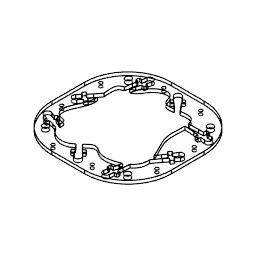
MidPlateShellBearing_v33 (Autodesk Fusion 360 design; units mm, degrees)
Autodesk Fusion 360 part; units mm, degrees
(part 1 of 2)
sketch "Sketch1" plane through (0, 0, 0) normal (0, 0, 1) x (1, 0, 0)
  line L0 (-33.4, -17.4) -> (-33.4, 33.4) construction
  line L1 (-33.4, 33.4) -> (-27.4, 33.4) construction
  line L2 (-33.4, -17.4) -> (-36.4, -17.4)
  line L3 (-36.4, -17.4) -> (-36.4, -27.4)
  line L4 (-36.4, -27.4) -> (-33.4, -27.4)
  line L5 (-33.4, -27.4) -> (-33.4, -17.4)
  line L6 (-27.4, 33.4) -> (-17.4, 33.4)
  line L7 (-17.4, 33.4) -> (-17.4, 36.4)
  line L8 (-17.4, 36.4) -> (-27.4, 36.4)
  line L9 (-27.4, 36.4) -> (-27.4, 33.4)
  line L10 (-17.4, 33.4) -> (33.4, 33.4) construction
  line L11 (33.4, 33.4) -> (33.4, 27.4) construction
  line L12 (33.4, 27.4) -> (36.4, 27.4)
  line L13 (36.4, 27.4) -> (36.4, 17.4)
  line L14 (36.4, 17.4) -> (33.4, 17.4)
  line L15 (33.4, 17.4) -> (33.4, 27.4)
  line L16 (33.4, 17.4) -> (33.4, -33.4) construction
  line L17 (33.4, -33.4) -> (27.4, -33.4) construction
  line L18 (27.4, -33.4) -> (17.4, -33.4)
  line L19 (17.4, -33.4) -> (17.4, -36.4)
  line L20 (17.4, -36.4) -> (27.4, -36.4)
  line L21 (27.4, -36.4) -> (27.4, -33.4)
  line L22 (17.4, -33.4) -> (-33.4, -33.4) construction
  line L23 (-33.4, -33.4) -> (-33.4, -27.4) construction
  line L24 (33.4, 33.4) -> (-33.4, -33.4) construction
  line L25 (33.4, -33.4) -> (-33.4, 33.4) construction
  line L26 (55, -55) -> (-55, -55)
  line L27 (-55, -55) -> (-55, 55)
  line L28 (-55, 55) -> (55, 55)
  line L29 (55, 55) -> (55, -55)
  line L30 (55, -55) -> (-55, 55) construction
  line L31 (-55, -55) -> (55, 55) construction
  line L32 (-34.9, -17.4) -> (-34.9, -7.75) construction
  line L33 (-34.9, -7.75) -> (-38.15, -7.75) construction
  circle A0 centre (-38.15, -7.75) radius 1.25
  line L34 (-34.9, -27.4) -> (-34.9, -38.15) construction
  line L35 (-34.9, -38.15) -> (-37.75, -38.15) construction
  circle A1 centre (-37.75, -38.15) radius 1.25
  circle A2 centre (38.15, -37.75) radius 1.25
  circle A3 centre (7.75, -38.15) radius 1.25
  circle A4 centre (37.75, 38.15) radius 1.25
  circle A5 centre (38.15, 7.75) radius 1.25
  circle A6 centre (-38.15, 37.75) radius 1.25
  circle A7 centre (-7.75, 38.15) radius 1.25
  constraint vertical L0
  constraint perpendicular L0 L1
  constraint horizontal L2
  constraint vertical L3
  constraint horizontal L4
  constraint vertical L5
  constraint horizontal L6
  constraint vertical L7
  constraint horizontal L8
  constraint vertical L9
  constraint perpendicular L7 L10
  constraint perpendicular L10 L11
  constraint horizontal L12
  constraint vertical L13
  constraint horizontal L14
  constraint vertical L15
  constraint perpendicular L14 L16
  constraint perpendicular L16 L17
  constraint horizontal L18
  constraint vertical L19
  constraint horizontal L20
  constraint vertical L21
  constraint perpendicular L19 L22
  constraint coincident origin L24
  constraint coincident origin L25
  constraint horizontal L26
  constraint perpendicular L26 L27
  constraint parallel L26 L28
  constraint parallel L27 L29
  constraint coincident L30 origin
  constraint coincident L31 origin
  constraint midpoint L2 L32.start
  constraint perpendicular L2 L32
  constraint perpendicular L32 L33
  constraint coincident L33.end A0.centre
  constraint midpoint L4 L34.start
  constraint perpendicular L4 L34
  constraint perpendicular L34 L35
  constraint coincident L35.end A1.centre
  measures "d1" distance of L0.start L0.end
  measures "d2" distance of L0.end L1.end
  measures "d3" distance of L0.start L2.end
  measures "d4" distance of L0.start L4.end
  measures "d5" distance of L1.end L6.end
  measures "d6" distance of L1.end L8.end
  measures "d7" distance of L6.end L10.end
  measures "d8" distance of L10.end L11.end
  measures "d9" distance of L11.end L12.end
  measures "d10" distance of L11.end L14.end
  measures "d11" distance of L14.end L16.end
  measures "d12" distance of L16.end L17.end
  measures "d13" distance of L17.end L18.end
  measures "d14" distance of L17.end L20.end
  measures "d15" distance of L18.end L22.end
  measures "d16" distance of L27.end L28.end
  measures "d17" distance of L26.end L27.end
  measures "d22" distance of L32.start L32.end
  measures "d23" distance of L32.end L33.end
  measures "d24" diameter of A0
  measures "d25" distance of L34.start L34.end
  measures "d26" distance of L34.end L35.end
  measures "d27" diameter of A1
extrude "Extrude1" add sketch "Sketch1" along normal blind 3 contours L2 L3 L4 L5 | L6 L7 L8 L9 | L12 L13 L14 L15 | L18 L19 L20 L21 | L26 L27 L28 L29 | A0 | A1 | A2 | A3 | A4 | A5 | A6 | A7
fillet "Fillet1" radius 40 4 edges at (-55, 55, 1.5) (55, 55, 1.5) (55, -55, 1.5) (-55, -55, 1.5)
other "Sketch1 (1)"
sketch "sketch 2514" plane through (0, 0, 0) normal (0, 0, 1) x (1, 0, 0)
  line L0 (55, -55) -> (-55, -55)
  line L1 (-55, -55) -> (-55, 55)
  line L2 (-55, 55) -> (55, 55)
  line L3 (55, 55) -> (55, -55)
  circle A0 centre (-27, 47) radius 3
  circle A1 centre (-1, 47) radius 3
  circle A2 centre (-47, -1) radius 3
  circle A3 centre (-47, -27) radius 3
  circle A4 centre (3.8268, 9.2388) radius 2.1
  line L4 (3.8268, 9.2388) -> (0, 0) construction
  circle A5 centre (-3.8268, 9.2388) radius 2.1
  circle A6 centre (-9.2388, 3.8268) radius 2.1
  circle A7 centre (-9.2388, -3.8268) radius 2.1
  circle A8 centre (-3.8268, -9.2388) radius 2.1
  circle A9 centre (3.8268, -9.2388) radius 2.1
  circle A10 centre (9.2388, -3.8268) radius 2.1
  circle A11 centre (9.2388, 3.8268) radius 2.1
  circle A12 centre (-47, -27) radius 3
  circle A13 centre (-47, -1) radius 3
  circle A14 centre (27, -47) radius 3
  circle A15 centre (1, -47) radius 3
  circle A16 centre (47, 27) radius 3
  circle A17 centre (47, 1) radius 3
  line L5 (3.8268, 9.2388) -> (-7.356, 51.4484) construction
  line L6 (-3.8267, 9.2387) -> (-39.1481, 32.3388) construction
  line L7 (-9.2241, 3.8302) -> (-38.1078, -2.8395) construction
  line L8 (-9.2387, -3.8268) -> (-45.7313, -32.4091) construction
  line L9 (-3.8418, -9.2572) -> (-24.5372, -34.632) construction
  line L10 (3.8268, -9.2388) -> (20.7131, -35.7055) construction
  line L11 (9.2388, -3.8268) -> (32.7897, -8.1449) construction
  line L12 (9.2388, 3.8268) -> (22.4195, 22.4675) construction
  line L13 (0, 0) -> (0, 3) construction
  line L14 (-38.1078, -2.8395) -> (1, -47) construction
  line L15 (32.7897, -8.1449) -> (27, -47) construction
  line L16 (20.7131, -35.7055) -> (47, 1) construction
  line L17 (-39.1481, 32.3388) -> (47, 27) construction
  line L18 (22.4195, 22.4675) -> (-1, 47) construction
  line L19 (-45.7313, -32.4091) -> (-27, 47) construction
  line L20 (-24.5372, -34.632) -> (-47, -27) construction
  line L21 (-7.356, 51.4484) -> (-47, -1) construction
  circle A18 centre (-26.9265, -6.4155) radius 6 construction
  circle A19 centre (-26.5529, -27.6103) radius 6 construction
  circle A20 centre (21, -25) radius 6 construction
  circle A21 centre (26, -13) radius 6 construction
  circle A22 centre (14.6683, 21.8979) radius 6 construction
  circle A23 centre (-10, 38) radius 6 construction
  circle A24 centre (-16.8843, 24.9475) radius 6 construction
  circle A25 centre (-35.9644, -17.138) radius 6 construction
  line L22 (-1.2763, 20.3008) -> (2.7836, 21.3764)
  line L23 (-1.2763, 20.3008) -> (1.7969, 8.701) construction
  line L24 (2.7836, 21.3764) -> (5.8568, 9.7766) construction
  line L25 (-15.0192, 14.0493) -> (-12.7204, 17.5644)
  line L26 (-20.4586, -0.9193) -> (-21.4036, 3.173)
  line L27 (-19.9809, -9.573) -> (-17.3911, -12.8795)
  line L28 (-13.0386, -17.2108) -> (-9.7838, -19.8654)
  line L29 (8.5109, -20.4847) -> (12.0516, -18.2256)
  line L30 (21.4208, -3.9254) -> (20.6633, -8.0565)
  line L31 (14.4523, 14.8373) -> (17.8816, 12.4124)
  line L32 (-12.7204, 17.5644) -> (-2.6774, 10.9963) construction
  line L33 (-15.0192, 14.0493) -> (-4.9762, 7.4813) construction
  line L34 (-21.4036, 3.173) -> (-9.7113, 5.873) construction
  line L35 (-20.4586, -0.9193) -> (-8.7663, 1.7807) construction
  line L36 (-19.9809, -9.573) -> (-10.5337, -2.1736) construction
  line L37 (-17.3911, -12.8795) -> (-7.9439, -5.4801) construction
  line L38 (-9.7838, -19.8654) -> (-2.1995, -10.5661) construction
  line L39 (-13.0386, -17.2108) -> (-5.4542, -7.9115) construction
  line L40 (12.0516, -18.2256) -> (5.5972, -8.1093) construction
  line L41 (8.5109, -20.4847) -> (2.0565, -10.3683) construction
  line L42 (20.6633, -8.0565) -> (8.8601, -5.8924) construction
  line L43 (21.4208, -3.9254) -> (9.6175, -1.7613) construction
  line L44 (14.4523, 14.8373) -> (7.5241, 5.0393) construction
  line L45 (17.8816, 12.4124) -> (10.9534, 2.6144) construction
  line L46 (26.6915, -34.8215) -> (30.8456, -35.4405)
  line L47 (-8.5279, -39.4086) -> (-5.3836, -36.6241)
  line L48 (-34.9623, -28.872) -> (-36.3135, -32.8488)
  line L49 (-41.4394, 9.8393) -> (-38.0888, 7.3067)
  line L50 (-31.7989, 35.8027) -> (-27.7111, 34.8384)
  line L51 (5.7671, 36.87) -> (8.8051, 39.7702)
  line L52 (35.1529, 29.8382) -> (34.8931, 25.6463)
  line L53 (38.3057, -7.5335) -> (41.7204, -9.9789)
  line L54 (30.8456, -35.4405) -> (29.9922, -47.2169)
  line L55 (26.6915, -34.8215) -> (24.0746, -46.3351)
  line L56 (-5.3836, -36.6241) -> (3.0893, -44.8472)
  line L57 (-8.5279, -39.4086) -> (-1.3897, -48.8137)
  line L58 (-34.9623, -28.872) -> (-45.8232, -24.2404)
  line L59 (-36.3135, -32.8488) -> (-47.7479, -29.9053)
  line L60 (-41.4394, 9.8393) -> (-49.2498, 0.9845)
  line L61 (-38.0888, 7.3067) -> (-44.477, -2.6231)
  line L62 (-27.7111, 34.8384) -> (-24.1405, 46.0928)
  line L63 (-31.7989, 35.8027) -> (-29.9635, 47.4663)
  line L64 (8.8051, 39.7702) -> (1.3202, 48.9018)
  line L65 (5.7671, 36.87) -> (-3.0074, 44.7706)
  line L66 (35.1529, 29.8382) -> (46.959, 29.9997)
  line L67 (34.8931, 25.6463) -> (46.5889, 24.0283)
  line L68 (41.7204, -9.9789) -> (49.3002, -0.9259)
  line L69 (38.3057, -7.5335) -> (44.436, 2.5576)
  circle A26 centre (-10, 38) radius 1.5
  circle A27 centre (-17, 25) radius 1.5
  circle A28 centre (14.6683, 21.8979) radius 1.5
  circle A29 centre (-26.9265, -6.4155) radius 1.5
  circle A30 centre (-36, -17) radius 1.5
  circle A31 centre (-26.5529, -27.6103) radius 1.5
  circle A32 centre (21, -25) radius 1.5
  circle A33 centre (26, -13) radius 1.5
  line L70 (-13.8698, 15.8068) -> (-3.8268, 9.2388) construction
  line L71 (0.7536, 20.8386) -> (3.8268, 9.2388) construction
  line L72 (9.2388, 3.8268) -> (16.1669, 13.6248) construction
  line L73 (9.2388, -3.8268) -> (21.042, -5.9909) construction
  line L74 (3.8268, -9.2388) -> (10.2813, -19.3551) construction
  line L75 (-3.8418, -9.2572) -> (-11.4112, -18.5381) construction
  line L76 (-9.2388, -3.8268) -> (-18.686, -11.2262) construction
  line L77 (-9.2241, 3.8302) -> (-20.9311, 1.1269) construction
  line L78 (-11.0342, 9.1729) -> (-6.6555, 15.8682) construction
  line L79 (-15.9776, 6.376) -> (-14.1776, -1.4189) construction
  line L80 (-16.4288, -4.3775) -> (-11.4959, -10.6756) construction
  line L81 (-10.7263, -11.3695) -> (-4.5268, -16.4258) construction
  line L82 (3.6819, -16.4484) -> (10.4262, -12.1455) construction
  line L83 (15.8618, -0.9745) -> (14.419, -8.8433) construction
  line L84 (9.4369, 11.0352) -> (15.9689, 6.4165) construction
  line L85 (-1.5764, 14.0143) -> (6.1568, 16.0631) construction
  line L86 (-7.9108, 16.6892) -> (-5.4001, 15.0472)
  line L87 (5.7727, 17.5131) -> (6.541, 14.6131)
  line L88 (-1.9605, 15.4643) -> (-1.1922, 12.5643)
  line L89 (-12.2895, 9.9939) -> (-9.7788, 8.3519)
  line L90 (-17.4391, 6.0385) -> (-14.516, 6.7135)
  line L91 (-15.6392, -1.7564) -> (-12.7161, -1.0814)
  line L92 (-17.6097, -5.3024) -> (-15.2479, -3.4525)
  line L93 (-12.6768, -11.6005) -> (-10.315, -9.7507)
  line L94 (-11.6743, -12.5319) -> (-9.7782, -10.2071)
  line L95 (-5.4748, -17.5882) -> (-3.5787, -15.2634)
  line L96 (2.8751, -15.1839) -> (4.4887, -17.713)
  line L97 (9.6194, -10.8809) -> (11.233, -13.41)
  line L98 (12.9436, -8.5728) -> (15.8945, -9.1138)
  line L99 (14.3864, -0.704) -> (17.3372, -1.245)
  line L100 (16.8349, 7.6412) -> (15.1028, 5.1917)
  line L101 (10.3029, 12.26) -> (8.5708, 9.8105)
  line L102 (5.7727, 17.5131) -> (3.9361, 17.0265)
  line L103 (6.541, 14.6131) -> (4.7044, 14.1265)
  line L104 (-1.9605, 15.4643) -> (-0.1239, 15.9509)
  line L105 (-1.1922, 12.5643) -> (0.6444, 13.0509)
  line L106 (-7.9108, 16.6892) -> (-8.8814, 15.0537)
  line L107 (-5.4001, 15.0472) -> (-6.4401, 13.4571)
  line L108 (-12.2895, 9.9939) -> (-11.2496, 11.584)
  line L109 (-9.7788, 8.3519) -> (-8.7389, 9.942)
  line L110 (-17.4391, 6.0385) -> (-17.0116, 4.1872)
  line L111 (-14.516, 6.7135) -> (-14.0886, 4.8622)
  line L112 (-12.7161, -1.0814) -> (-13.1436, 0.7699)
  line L113 (-15.6392, -1.7564) -> (-16.0666, 0.0949)
  line L114 (-15.2479, -3.4525) -> (-14.0764, -4.9483)
  line L115 (-17.6097, -5.3024) -> (-16.4382, -6.7982)
  line L116 (-10.315, -9.7507) -> (-11.4866, -8.2549)
  line L117 (-12.6768, -11.6005) -> (-13.8484, -10.1047)
  line L118 (-9.7782, -10.2071) -> (-8.3058, -11.408)
  line L119 (-11.6743, -12.5319) -> (-10.2019, -13.7328)
  line L120 (-3.5787, -15.2634) -> (-5.0511, -14.0625)
  line L121 (-5.4748, -17.5882) -> (-6.9472, -16.3873)
  line L122 (2.8751, -15.1839) -> (4.4769, -14.1619)
  line L123 (4.4887, -17.713) -> (6.0905, -16.691)
  line L124 (11.233, -13.41) -> (9.6312, -14.432)
  line L125 (9.6194, -10.8809) -> (8.0176, -11.9029)
  line L126 (15.8945, -9.1138) -> (16.2371, -7.245)
  line L127 (12.9436, -8.5728) -> (13.2863, -6.7039)
  line L128 (17.3372, -1.245) -> (16.9945, -3.1138)
  line L129 (14.3864, -0.704) -> (14.0437, -2.5728)
  line L130 (16.8349, 7.6412) -> (15.2835, 8.7382)
  line L131 (15.1028, 5.1917) -> (13.5515, 6.2887)
  line L132 (8.5708, 9.8105) -> (10.1222, 8.7135)
  line L133 (10.3029, 12.26) -> (11.8542, 11.163)
  line L134 (-6.9558, -38.0164) -> (1, -47) construction
  line L135 (27, -47) -> (28.7686, -35.131) construction
  line L136 (47, 1) -> (40.0131, -8.7562) construction
  line L137 (47, 27) -> (35.023, 27.7422) construction
  line L138 (-1, 47) -> (7.2861, 38.3201) construction
  line L139 (-27, 47) -> (-29.755, 35.3205) construction
  line L140 (-47, -1) -> (-39.7641, 8.573) construction
  line L141 (-47, -27) -> (-35.6379, -30.8604) construction
  line L142 (-6.7211, -45.8231) -> (0.7653, -39.1933) construction
  line L143 (22.9389, -40.3286) -> (32.8297, -41.8024) construction
  line L144 (39.4415, -0.9669) -> (47.5716, -6.7893) construction
  line L145 (41.3208, 32.3615) -> (40.7022, 22.3807) construction
  line L146 (-0.4736, 39.2075) -> (6.7597, 46.1126) construction
  line L147 (-33.2439, 42.3082) -> (-23.511, 40.0124) construction
  line L148 (-47.3708, 6.8014) -> (-39.3933, 0.7715) construction
  line L149 (-39.7105, -24.196) -> (-42.9275, -33.6644) construction
  line L150 (-7.7155, -44.7001) -> (-5.7266, -46.946)
  line L151 (-0.2292, -38.0703) -> (1.7598, -40.3162)
  line L152 (23.16, -38.845) -> (22.7178, -41.8122)
  line L153 (33.0508, -40.3188) -> (32.6086, -43.286)
  line L154 (38.5681, -2.1864) -> (40.3148, 0.2527)
  line L155 (46.6982, -8.0088) -> (48.445, -5.5698)
  line L156 (39.2051, 22.4735) -> (42.1994, 22.2879)
  line L157 (39.8236, 32.4543) -> (42.8179, 32.2688)
  line L158 (-1.5093, 40.2925) -> (0.5622, 38.1225)
  line L159 (5.7239, 47.1976) -> (7.7954, 45.0276)
  line L160 (-32.8996, 43.7681) -> (-33.5883, 40.8482)
  line L161 (-23.8554, 38.5524) -> (-23.1667, 41.4723)
  line L162 (-48.2753, 5.6048) -> (-46.4663, 7.9981)
  line L163 (-40.2978, -0.4251) -> (-38.4888, 1.9682)
  line L164 (-41.1307, -23.7134) -> (-38.2902, -24.6785)
  line L165 (-44.3477, -33.1819) -> (-41.5072, -34.147)
  line L166 (-7.7155, -44.7001) -> (-5.7996, -43.0034)
  line L167 (-5.7266, -46.946) -> (-3.9807, -45.3999)
  line L168 (-0.2292, -38.0703) -> (-2.1451, -39.7671)
  line L169 (1.7598, -40.3162) -> (0.0138, -41.8624)
  line L170 (23.16, -38.845) -> (25.6913, -39.2222)
  line L171 (22.7178, -41.8122) -> (25.0245, -42.156)
  line L172 (33.0508, -40.3188) -> (30.5194, -39.9416)
  line L173 (32.6086, -43.286) -> (30.3019, -42.9423)
  line L174 (40.3148, 0.2527) -> (42.2109, -1.1052)
  line L175 (38.5681, -2.1864) -> (40.6488, -3.6765)
  line L176 (48.445, -5.5698) -> (46.5489, -4.2119)
  line L177 (46.6982, -8.0088) -> (44.6175, -6.5187)
  line L178 (39.8236, 32.4543) -> (39.6653, 29.8999)
  line L179 (42.8179, 32.2688) -> (42.6736, 29.9411)
  line L180 (42.1994, 22.2879) -> (42.3436, 24.6156)
  line L181 (39.2051, 22.4735) -> (39.3634, 25.0279)
  line L182 (-1.5093, 40.2925) -> (0.1776, 41.9029)
  line L183 (0.5622, 38.1225) -> (2.4134, 39.8897)
  line L184 (7.7954, 45.0276) -> (5.9442, 43.2604)
  line L185 (5.7239, 47.1976) -> (4.037, 45.5872)
  line L186 (-32.8996, 43.7681) -> (-30.6297, 43.2327)
  line L187 (-33.5883, 40.8482) -> (-31.0974, 40.2607)
  line L188 (-23.1667, 41.4723) -> (-25.4365, 42.0077)
  line L189 (-23.8554, 38.5524) -> (-26.3463, 39.14)
  line L190 (-46.4663, 7.9981) -> (-44.4246, 6.4548)
  line L191 (-48.2753, 5.6048) -> (-46.4148, 4.1986)
  line L192 (-38.4888, 1.9682) -> (-40.5305, 3.5114)
  line L193 (-40.2978, -0.4251) -> (-42.1583, 0.9812)
  line L194 (-38.2902, -24.6785) -> (-39.1135, -27.1018)
  line L195 (-41.1307, -23.7134) -> (-41.881, -25.9216)
  line L196 (-41.5072, -34.147) -> (-40.6839, -31.7237)
  line L197 (-44.3477, -33.1819) -> (-43.5975, -30.9737)
  line L198 (1, -47) -> (27, -47) construction
  line L199 (-47, -1) -> (-47, -27) construction
  line L200 (47, 1) -> (47, 27) construction
  line L201 (-1, 47) -> (-27, 47) construction
  circle A34 centre (14, -47) radius 1.5
  circle A35 centre (-47, -14) radius 1.5
  circle A36 centre (47, 14) radius 1.5
  circle A37 centre (-14, 47) radius 1.5
  circle A38 centre (0, 0) radius 6
  line L202 (-15.5118, 13.2961) -> (-12.2278, 18.3176)
  line L203 (-21.6061, 4.0499) -> (-20.2561, -1.7962)
  line L204 (-20.5358, -8.8644) -> (-16.8361, -13.588)
  line L205 (-13.736, -16.642) -> (-9.0864, -20.4342)
  line L206 (7.7522, -20.9687) -> (12.8103, -17.7415)
  line L207 (20.501, -8.9418) -> (21.5831, -3.0401)
  line L208 (13.7174, 15.3569) -> (18.6164, 11.8928)
  line L209 (-2.1463, 20.0703) -> (3.6536, 21.6069)
  line L210 (1.7969, 8.701) -> (-2.1463, 20.0703)
  line L211 (3.6536, 21.6069) -> (5.8568, 9.7766)
  line L212 (13.7174, 15.3569) -> (7.4388, 4.9085)
  line L213 (18.6164, 11.8928) -> (10.9534, 2.6144)
  line L214 (21.5831, -3.0401) -> (9.6175, -1.7613)
  line L215 (20.501, -8.9418) -> (8.8601, -5.8924)
  line L216 (12.8103, -17.7415) -> (5.5972, -8.1093)
  line L217 (7.7522, -20.9687) -> (2.0565, -10.3683)
  line L218 (-13.736, -16.642) -> (-5.4542, -7.9115)
  line L219 (-9.0864, -20.4342) -> (-2.1995, -10.5661)
  line L220 (-20.5358, -8.8644) -> (-10.5337, -2.1736)
  line L221 (-16.8361, -13.588) -> (-7.9439, -5.4801)
  line L222 (-21.6061, 4.0499) -> (-9.7113, 5.873)
  line L223 (-20.2561, -1.7962) -> (-8.6156, 1.8214)
  line L224 (-15.5118, 13.2961) -> (-4.8425, 7.4007)
  line L225 (-12.2278, 18.3176) -> (-2.6774, 10.9963)
  point P0 (0.7536, 20.8386)
  point P1 (-13.8698, 15.8068)
  point P2 (-20.9311, 1.1269)
  point P3 (-18.686, -11.2262)
  point P4 (-11.4112, -18.5381)
  point P5 (10.2813, -19.3551)
  point P6 (21.042, -5.9909)
  point P7 (16.1669, 13.6248)
  point P8 (28.7686, -35.131)
  point P9 (-6.9558, -38.0164)
  point P10 (-35.6379, -30.8604)
  point P11 (-39.7641, 8.573)
  point P12 (-29.755, 35.3205)
  point P13 (7.2861, 38.3201)
  point P14 (35.023, 27.7422)
  point P15 (40.0131, -8.7562)
  point P16 (-8.8448, 12.5205)
  point P17 (-15.0776, 2.4786)
  point P18 (-13.9624, -7.5265)
  point P19 (-7.6265, -13.8976)
  point P20 (7.054, -14.297)
  point P21 (15.1404, -4.9089)
  point P22 (12.7029, 8.7258)
  point P23 (2.2902, 15.0387)
  point P24 (-2.9779, -42.5082)
  point P25 (27.8843, -41.0655)
  point P26 (43.5065, -3.8781)
  point P27 (41.0115, 27.3711)
  point P28 (3.1431, 42.6601)
  point P29 (-28.3775, 41.1603)
  point P30 (-43.3821, 3.7865)
  point P31 (-41.319, -28.9302)
extrude "Extrude6" cut sketch "sketch 2514" along normal blind 9 contours A0 | A0 L50 L62 L63 | L63 L160 L186 L187 | L62 L161 L188 L189 | A1 | A1 L51 L64 L65 | L64 L159 L184 L185 | L65 L158 L182 L183 | A2 A13 | A2 A13 L49 L60 L61 | L60 L162 L190 L191 | L61 L163 L192 L193 | A3 A12 | A3 A12 L48 L58 L59 | L58 L164 L194 L195 | L59 L165 L196 L197 | A14 | A14 L46 L54 L55 | L55 L152 L170 L171 | L54 L153 L172 L173 | A15 | A15 L47 L56 L57 | L56 L151 L168 L169 | L57 L150 L166 L167 | A16 | A16 L52 L66 L67 | L66 L157 L178 L179 | L67 L156 L180 L181 | A17 | A17 L53 L68 L69 | L69 L154 L174 L175 | L68 L155 L176 L177
other "Sketch1 (2)"
extrude "Extrude9" cut sketch "sketch 2514" along normal blind 15 contours A34 | A35 | A36 | A37
other "Sketch7"
sketch "sketch 8346" plane through (0, 0, 0) normal (0, 0, -1) x (1, 0, 0)
  arc A0 (-15, 55) -> (-55, 15) centre (-15, 15) ccw
  line L0 (-55, 15) -> (-55, -15)
  arc A1 (-55, -15) -> (-15, -55) centre (-15, -15) ccw
  line L1 (-15, -55) -> (15, -55)
  arc A2 (15, -55) -> (55, -15) centre (15, -15) ccw
  line L2 (55, -15) -> (55, 15)
  arc A3 (55, 15) -> (15, 55) centre (15, 15) ccw
  line L3 (15, 55) -> (-15, 55)
  line L4 (30.8456, 35.4405) -> (26.6915, 34.8215)
  line L5 (26.6915, 34.8215) -> (24.0746, 46.3351)
  arc A4 (29.9922, 47.2169) -> (24.0746, 46.3351) centre (27, 47) ccw
  line L6 (29.9922, 47.2169) -> (30.8456, 35.4405)
  arc A5 (-3.0074, -44.7706) -> (1.3202, -48.9018) centre (-1, -47) ccw
  line L7 (-3.0074, -44.7706) -> (5.7671, -36.87)
  line L8 (5.7671, -36.87) -> (8.8051, -39.7702)
  line L9 (8.8051, -39.7702) -> (1.3202, -48.9018)
  line L10 (-36.3135, 32.8488) -> (-34.9623, 28.872)
  line L11 (-34.9623, 28.872) -> (-45.8232, 24.2404)
  arc A6 (-47.7479, 29.9053) -> (-45.8232, 24.2404) centre (-47, 27) ccw
  line L12 (-47.7479, 29.9053) -> (-36.3135, 32.8488)
  arc A7 (46.959, -29.9997) -> (46.5889, -24.0283) centre (47, -27) ccw
  line L13 (46.959, -29.9997) -> (35.1529, -29.8382)
  line L14 (35.1529, -29.8382) -> (34.8931, -25.6463)
  line L15 (34.8931, -25.6463) -> (46.5889, -24.0283)
  line L16 (-5.3836, 36.6241) -> (-8.5279, 39.4086)
  line L17 (-8.5279, 39.4086) -> (-1.3897, 48.8137)
  arc A8 (3.0893, 44.8472) -> (-1.3897, 48.8137) centre (1, 47) ccw
  line L18 (3.0893, 44.8472) -> (-5.3836, 36.6241)
  arc A9 (-29.9635, -47.4663) -> (-24.1405, -46.0928) centre (-27, -47) ccw
  line L19 (-29.9635, -47.4663) -> (-31.7989, -35.8027)
  line L20 (-31.7989, -35.8027) -> (-27.7111, -34.8384)
  line L21 (-27.7111, -34.8384) -> (-24.1405, -46.0928)
  line L22 (-38.0888, -7.3067) -> (-41.4394, -9.8393)
  line L23 (-41.4394, -9.8393) -> (-49.2498, -0.9845)
  arc A10 (-44.477, 2.6231) -> (-49.2498, -0.9845) centre (-47, 1) ccw
  line L24 (-44.477, 2.6231) -> (-38.0888, -7.3067)
  arc A11 (44.436, -2.5576) -> (49.3002, 0.9259) centre (47, -1) ccw
  line L25 (44.436, -2.5576) -> (38.3057, 7.5335)
  line L26 (38.3057, 7.5335) -> (41.7204, 9.9789)
  line L27 (41.7204, 9.9789) -> (49.3002, 0.9259)
  spline S0 degree 5 poles (6, 33) (5.6161, 32.7729) (4.8585, 32.3129) (3.7455, 31.6318) (2.2849, 30.8699) (0.452, 30.4996) (-1.4333, 30.9701) (-3.4282, 32.3455) (-5.6081, 34.431) (-8.0444, 36.8766) (-10.7879, 39.2518) (-13.8487, 41.1342) (-17.1801, 42.1877) (-20.6559, 42.2545) (-24.0634, 41.4126) (-27.158, 39.8834) (-29.7084, 37.9638) (-31.5485, 35.9438) (-32.6181, 34.0418) (-33.0288, 32.3038) (-33.0424, 30.6287) (-32.9614, 28.915) (-33.0417, 27.1834) (-33.403, 25.6896) (-34.0832, 24.7061) (-35.0951, 24.2854) (-36.458, 24.1219) (-38.1353, 23.8108) (-39.9672, 23.09) (-41.7048, 21.8735) (-43.0907, 20.1791) (-43.9235, 18.0916) (-44.1323, 15.7105) (-43.7511, 13.1365) (-42.8906, 10.4563) (-41.7112, 7.7293) (-40.3948, 4.9709) (-39.1191, 2.1444) (-38.0419, -0.8122) (-37.284, -3.9616) (-36.913, -7.3428) (-36.9262, -10.9459) (-37.2348, -14.688) (-37.6458, -18.3876) (-37.9149, -21.8152) (-37.7966, -24.7431) (-37.0987, -26.9971) (-35.7287, -28.5033) (-33.7572, -29.3478) (-31.4338, -29.7956) (-29.07, -30.1864) (-26.9454, -30.8538) (-25.2054, -32.0348) (-23.7602, -33.782) (-22.3771, -36.0014) (-20.7773, -38.4934) (-18.7331, -40.9922) (-16.16, -43.2063) (-13.223, -44.8582) (-10.239, -45.7206) (-7.5648, -45.6503) (-5.4874, -44.6253) (-4.1211, -42.776) (-3.2794, -40.4321) (-2.573, -38.036) (-1.5546, -36.0287) (0.163, -34.7542) (2.7522, -34.333) (6.1232, -34.6309) (10.02, -35.3552) (14.0819, -36.1205) (17.9195, -36.5264) (21.1833, -36.2308) (23.6364, -35.0241) (25.2257, -32.904) (26.0383, -30.0178) (26.259, -26.6039) (26.1252, -22.9326) (25.8856, -19.251) (25.7518, -15.7155) (25.8753, -12.3728) (26.3531, -9.1972) (27.2263, -6.1141) (28.4811, -3.0276) (30.049, 0.1527) (31.8071, 3.4845) (33.5791, 6.9674) (35.16, 10.5574) (36.3393, 14.1786) (36.9248, 17.7364) (36.7669, 21.1302) (35.7804, 24.2655) (33.9723, 27.0679) (31.454, 29.4919) (28.4049, 31.5128) (25.0439, 33.1212) (21.5976, 34.3174) (18.2695, 35.104) (15.2109, 35.482) (12.4848, 35.4406) (10.0799, 34.9794) (8.3661, 34.3055) (7.1618, 33.6757) (6.3839, 33.2271) (6, 33) knots 0 0 0 0 0 0 0.01 0.02 0.03 0.04 0.05 0.06 0.07 0.08 0.09 0.1 0.11 0.12 0.13 0.14 0.15 0.16 0.17 0.18 0.19 0.2 0.21 0.22 0.23 0.24 0.25 0.26 0.27 0.28 0.29 0.3 0.31 0.32 0.33 0.34 0.35 0.36 0.37 0.38 0.39 0.4 0.41 0.42 0.43 0.44 0.45 0.46 0.47 0.48 0.49 0.5 0.51 0.52 0.53 0.54 0.55 0.56 0.57 0.58 0.59 0.6 0.61 0.62 0.63 0.64 0.65 0.66 0.67 0.68 0.69 0.7 0.71 0.72 0.73 0.74 0.75 0.76 0.77 0.78 0.79 0.8 0.81 0.82 0.83 0.84 0.85 0.86 0.87 0.88 0.89 0.9 0.91 0.92 0.93 0.94 0.95 0.96 0.97 0.98 0.99 1 1 1 1 1 1
  line L28 (-31.7989, -35.8027) -> (-32.7908, -29.4916)
  line L29 (-27.7111, -34.8384) -> (-28.7703, -30.3481)
  line L30 (5.7671, -36.87) -> (7.6106, -34.9389)
  line L31 (8.8051, -39.7702) -> (12.1168, -35.7299)
  line L32 (34.8931, -25.6463) -> (26.1751, -26.1865)
  line L33 (35.1529, -29.8382) -> (25.9192, -29.7135)
  line L34 (41.7204, 9.9789) -> (36.6853, 17.0096)
  line L35 (38.3057, 7.5335) -> (35.421, 11.5615)
  line L36 (26.6915, 34.8215) -> (27.102, 32.0663)
  line L37 (30.8456, 35.4405) -> (31.2814, 29.4234)
  line L38 (-5.3836, 36.6241) -> (-6.5195, 35.3415)
  line L39 (-8.5279, 39.4086) -> (-9.6251, 38.1696)
  line L40 (-36.3135, 32.8488) -> (-32.416, 34.173)
  line L41 (-34.9623, 28.872) -> (-33.0026, 29.5379)
  line L42 (-38.0888, -7.3067) -> (-36.9644, -8.7943)
  line L43 (-41.4394, -9.8393) -> (-37.3179, -15.2919)
  point P0 (-1, 31)
  point P1 (-16.538, 41.8122)
  point P2 (-32, 35)
  point P3 (-33, 29)
  point P4 (-34, 25)
  point P5 (-37, 24)
  point P6 (-43, 20)
  point P7 (-41.881, 8.1792)
  point P8 (-37, -11)
  point P9 (-36, -28)
  point P10 (-27, -31)
  point P11 (-18.417, -41.1068)
  point P12 (-5.3903, -44.1795)
  point P13 (-0.4567, -35.3941)
  point P14 (21, -36)
  point P15 (26, -21)
  point P16 (30, 0)
  point P17 (35.8821, 23.4737)
  point P18 (17.6572, 35.1174)
extrude "Extrude10" cut sketch "sketch 8346" against normal blind 50 contours L4 S0 L36 L37 | S0 | L26 S0 L34 L35 | L16 S0 L38 L39 | L14 S0 L32 L33 | L10 S0 L40 L41 | L8 S0 L30 L31 | L22 S0 L42 L43 | L20 S0 L28 L29
sketch "Sketch4" plane through (0, 0, 3) normal (0, 0, 1) x (-1, 0, 0)
  circle A0 centre (14, -47) radius 1.5
  circle A1 centre (-47, -14) radius 1.5
  circle A2 centre (47, 14) radius 1.5
  circle A3 centre (-14, 47) radius 1.5
  line L0 (41.4394, -9.8393) -> (37.3179, -15.2919)
  spline S0 degree 3 poles (37.3179, -15.2919) (37.6885, -19.157) (38.1371, -22.7222) (37.3203, -26.0559) (37.037, -26.7219) (36.2871, -27.772) (35.8641, -28.165) (34.6133, -28.9678) (33.7328, -29.2635) (32.7908, -29.4916) knots 0 0 0 0 1.164828 1.164828 1.516946 1.516946 1.81941 1.81941 2.270031 2.270031 2.270031 2.270031
  line L1 (32.7908, -29.4916) -> (31.7989, -35.8027)
  line L2 (31.7989, -35.8027) -> (31.0974, -40.2607)
  line L3 (31.0974, -40.2607) -> (33.5883, -40.8482)
  line L4 (33.5883, -40.8482) -> (32.8996, -43.7681)
  line L5 (32.8996, -43.7681) -> (30.6297, -43.2327)
  line L6 (30.6297, -43.2327) -> (29.9635, -47.4663)
  arc A4 (24.1405, -46.0928) -> (29.9635, -47.4663) centre (27, -47) ccw
  line L7 (24.1405, -46.0928) -> (25.4365, -42.0077)
  line L8 (25.4365, -42.0077) -> (23.1667, -41.4723)
  line L9 (23.1667, -41.4723) -> (23.8554, -38.5524)
  line L10 (23.8554, -38.5524) -> (26.3463, -39.14)
  line L11 (26.3463, -39.14) -> (27.7111, -34.8384)
  line L12 (27.7111, -34.8384) -> (28.7703, -30.3481)
  spline S1 degree 3 poles (28.7703, -30.3481) (27.6148, -30.6643) (26.6336, -31.0889) (24.9398, -32.4102) (24.298, -33.1659) (22.092, -36.2546) (20.5653, -39.283) (15.8311, -43.4069) (14.0247, -44.4113) (11.1819, -45.3972) (9.9898, -45.607) (8.1404, -45.5368) (7.3989, -45.3892) (6.1398, -44.8148) (5.64, -44.4531) (4.7208, -43.4815) (4.3496, -42.8831) (3.4629, -41.0501) (3.1013, -39.695) (2.3137, -37.6472) (1.9455, -36.8825) (1.0366, -35.7978) (0.5937, -35.4393) (-0.469, -34.89) (-1.0783, -34.7097) (-3.396, -34.3697) (-5.3987, -34.5812) (-7.6106, -34.9389) knots 0 0 0 0 0.359374 0.359374 0.670478 0.670478 1.446599 1.446599 1.895417 1.895417 2.224922 2.224922 2.450473 2.450473 2.63972 2.63972 2.850158 2.850158 3.247941 3.247941 3.519478 3.519478 3.715617 3.715617 3.915643 3.915643 4.385468 4.385468 4.385468 4.385468
  line L13 (-7.6106, -34.9389) -> (-5.7671, -36.87)
  line L14 (-5.7671, -36.87) -> (-2.4134, -39.8897)
  line L15 (-2.4134, -39.8897) -> (-0.5622, -38.1225)
  line L16 (-0.5622, -38.1225) -> (1.5093, -40.2925)
  line L17 (1.5093, -40.2925) -> (-0.1776, -41.9029)
  line L18 (-0.1776, -41.9029) -> (3.0074, -44.7706)
  arc A5 (-1.3202, -48.9018) -> (3.0074, -44.7706) centre (1, -47) ccw
  line L19 (-1.3202, -48.9018) -> (-4.037, -45.5872)
  line L20 (-4.037, -45.5872) -> (-5.7239, -47.1976)
  line L21 (-5.7239, -47.1976) -> (-7.7954, -45.0276)
  line L22 (-7.7954, -45.0276) -> (-5.9442, -43.2604)
  line L23 (-5.9442, -43.2604) -> (-12.1168, -35.7299)
  spline S2 degree 3 poles (-12.1168, -35.7299) (-14.7803, -36.1844) (-17.4077, -36.5262) (-20.6177, -36.1408) (-21.5954, -35.8949) (-23.1516, -35.0659) (-23.7332, -34.592) (-24.6878, -33.4235) (-25.0394, -32.7732) (-25.5995, -31.3254) (-25.7916, -30.5154) (-25.9192, -29.7135) knots 0 0 0 0 0.810588 0.810588 1.168868 1.168868 1.446193 1.446193 1.71283 1.71283 2.006296 2.006296 2.006296 2.006296
  line L24 (-25.9192, -29.7135) -> (-35.1529, -29.8382)
  line L25 (-35.1529, -29.8382) -> (-39.6653, -29.8999)
  line L26 (-39.6653, -29.8999) -> (-39.8236, -32.4543)
  line L27 (-39.8236, -32.4543) -> (-42.8179, -32.2688)
  line L28 (-42.8179, -32.2688) -> (-42.6736, -29.9411)
  line L29 (-42.6736, -29.9411) -> (-46.959, -29.9997)
  arc A6 (-46.5889, -24.0283) -> (-46.959, -29.9997) centre (-47, -27) ccw
  line L30 (-46.5889, -24.0283) -> (-42.3436, -24.6156)
  line L31 (-42.3436, -24.6156) -> (-42.1994, -22.2879)
  line L32 (-42.1994, -22.2879) -> (-39.2051, -22.4735)
  line L33 (-39.2051, -22.4735) -> (-39.3634, -25.0279)
  line L34 (-39.3634, -25.0279) -> (-34.8931, -25.6463)
  line L35 (-34.8931, -25.6463) -> (-26.1751, -26.1865)
  spline S3 degree 3 poles (-26.1751, -26.1865) (-26.2136, -21.5897) (-25.4228, -16.5889) (-26.5447, -7.6817) (-27.7362, -4.5994) (-31.4465, 2.9635) (-33.9112, 7.1935) (-35.421, 11.5615) knots 0 0 0 0 1.379101 1.379101 2.416171 2.416171 3.558045 3.558045 3.558045 3.558045
  line L36 (-35.421, 11.5615) -> (-38.3057, 7.5335)
  line L37 (-38.3057, 7.5335) -> (-40.6488, 3.6765)
  line L38 (-40.6488, 3.6765) -> (-38.5681, 2.1864)
  line L39 (-38.5681, 2.1864) -> (-40.3148, -0.2527)
  line L40 (-40.3148, -0.2527) -> (-42.2109, 1.1052)
  line L41 (-42.2109, 1.1052) -> (-44.436, -2.5576)
  arc A7 (-49.3002, 0.9259) -> (-44.436, -2.5576) centre (-47, -1) ccw
  line L42 (-49.3002, 0.9259) -> (-46.5489, 4.2119)
  line L43 (-46.5489, 4.2119) -> (-48.445, 5.5698)
  line L44 (-48.445, 5.5698) -> (-46.6982, 8.0088)
  line L45 (-46.6982, 8.0088) -> (-44.6175, 6.5187)
  line L46 (-44.6175, 6.5187) -> (-41.7204, 9.9789)
  line L47 (-41.7204, 9.9789) -> (-36.6853, 17.0096)
  spline S4 degree 3 poles (-36.6853, 17.0096) (-36.8676, 18.8531) (-36.7596, 20.6853) (-35.8249, 23.83) (-35.1927, 25.0859) (-33.4931, 27.4447) (-32.4383, 28.4998) (-31.2814, 29.4234) knots 0 0 0 0 0.555731 0.555731 0.983651 0.983651 1.42815 1.42815 1.42815 1.42815
  line L48 (-31.2814, 29.4234) -> (-30.8456, 35.4405)
  line L49 (-30.8456, 35.4405) -> (-30.5194, 39.9416)
  line L50 (-30.5194, 39.9416) -> (-33.0508, 40.3188)
  line L51 (-33.0508, 40.3188) -> (-32.6086, 43.286)
  line L52 (-32.6086, 43.286) -> (-30.3019, 42.9423)
  line L53 (-30.3019, 42.9423) -> (-29.9922, 47.2169)
  arc A8 (-24.0746, 46.3351) -> (-29.9922, 47.2169) centre (-27, 47) ccw
  line L54 (-24.0746, 46.3351) -> (-25.0245, 42.156)
  line L55 (-25.0245, 42.156) -> (-22.7178, 41.8122)
  line L56 (-22.7178, 41.8122) -> (-23.16, 38.845)
  line L57 (-23.16, 38.845) -> (-25.6913, 39.2222)
  line L58 (-25.6913, 39.2222) -> (-26.6915, 34.8215)
  line L59 (-26.6915, 34.8215) -> (-27.102, 32.0663)
  spline S5 degree 3 poles (-27.102, 32.0663) (-23.8561, 33.7038) (-20.1727, 34.7945) (-13.9908, 35.6095) (-11.9033, 35.3478) (-8.6393, 34.4929) (-7.241, 33.737) (-4.6779, 32.215) (-3.539, 31.4712) (-1.7666, 30.8258) (-1.1355, 30.6903) (0.1203, 30.7222) (0.6844, 30.8607) (1.9595, 31.399) (2.6674, 31.8714) (4.3852, 33.2548) (5.4117, 34.2687) (6.5195, 35.3415) knots 0 0 0 0 1.090679 1.090679 2.116632 2.116632 3.315493 3.315493 4.459674 4.459674 5.071625 5.071625 5.626071 5.626071 6.359803 6.359803 7.369828 7.369828 7.369828 7.369828
  line L60 (6.5195, 35.3415) -> (5.3836, 36.6241)
  line L61 (5.3836, 36.6241) -> (2.1451, 39.7671)
  line L62 (2.1451, 39.7671) -> (0.2292, 38.0703)
  line L63 (0.2292, 38.0703) -> (-1.7598, 40.3162)
  line L64 (-1.7598, 40.3162) -> (-0.0138, 41.8624)
  line L65 (-0.0138, 41.8624) -> (-3.0893, 44.8472)
  arc A9 (1.3897, 48.8137) -> (-3.0893, 44.8472) centre (-1, 47) ccw
  line L66 (1.3897, 48.8137) -> (3.9807, 45.3999)
  line L67 (3.9807, 45.3999) -> (5.7266, 46.946)
  line L68 (5.7266, 46.946) -> (7.7155, 44.7001)
  line L69 (7.7155, 44.7001) -> (5.7996, 43.0034)
  line L70 (5.7996, 43.0034) -> (8.5279, 39.4086)
  line L71 (8.5279, 39.4086) -> (9.6251, 38.1696)
  spline S6 degree 3 poles (9.6251, 38.1696) (11.2124, 39.4725) (12.9202, 40.5975) (16.4323, 41.9003) (18.0613, 42.1653) (21.4266, 42.0265) (23.0731, 41.6295) (26.5653, 40.2029) (28.3145, 39.0547) (30.2985, 37.2379) (30.8783, 36.6163) (31.7822, 35.4004) (32.1434, 34.8061) (32.416, 34.173) knots 0 0 0 0 0.616058 0.616058 1.127035 1.127035 1.633478 1.633478 2.269407 2.269407 2.553154 2.553154 2.787926 2.787926 2.787926 2.787926
  line L72 (32.416, 34.173) -> (36.3135, 32.8488)
  line L73 (36.3135, 32.8488) -> (40.6839, 31.7237)
  line L74 (40.6839, 31.7237) -> (41.5072, 34.147)
  line L75 (41.5072, 34.147) -> (44.3477, 33.1819)
  line L76 (44.3477, 33.1819) -> (43.5975, 30.9737)
  line L77 (43.5975, 30.9737) -> (47.7479, 29.9053)
  arc A10 (45.8232, 24.2404) -> (47.7479, 29.9053) centre (47, 27) ccw
  line L78 (45.8232, 24.2404) -> (41.881, 25.9216)
  line L79 (41.881, 25.9216) -> (41.1307, 23.7134)
  line L80 (41.1307, 23.7134) -> (38.2902, 24.6785)
  line L81 (38.2902, 24.6785) -> (39.1135, 27.1018)
  line L82 (39.1135, 27.1018) -> (34.9623, 28.872)
  line L83 (34.9623, 28.872) -> (33.0026, 29.5379)
  spline S7 degree 3 poles (33.0026, 29.5379) (32.9902, 28.5579) (33.003, 27.1751) (33.5348, 25.6326) (33.7207, 25.3268) (34.1024, 24.8702) (34.3236, 24.7044) (34.8418, 24.4372) (35.1527, 24.347) (36.4443, 24.0711) (37.7665, 23.9707) (40.2586, 22.8614) (41.1591, 22.2488) (42.5804, 20.7638) (43.1055, 19.9446) (43.8206, 18.0888) (43.9818, 17.0988) (44.0027, 14.699) (43.7263, 13.2998) (42.5231, 9.2938) (41.1447, 6.638) (39.093, 2.0196) (38.3333, 0.1029) (37.2326, -4.3021) (36.9907, -6.4921) (36.9644, -8.7943) knots 0 0 0 0 0.294006 0.294006 0.417435 0.417435 0.550082 0.550082 0.704478 0.704478 1.129194 1.129194 1.408869 1.408869 1.66214 1.66214 1.922723 1.922723 2.2812 2.2812 3.001747 3.001747 3.492602 3.492602 4.002499 4.002499 4.002499 4.002499
  line L84 (36.9644, -8.7943) -> (38.0888, -7.3067)
  line L85 (38.0888, -7.3067) -> (40.5305, -3.5114)
  line L86 (40.5305, -3.5114) -> (38.4888, -1.9682)
  line L87 (38.4888, -1.9682) -> (40.2978, 0.4251)
  line L88 (40.2978, 0.4251) -> (42.1583, -0.9812)
  line L89 (42.1583, -0.9812) -> (44.477, 2.6231)
  arc A11 (49.2498, -0.9845) -> (44.477, 2.6231) centre (47, 1) ccw
  line L90 (49.2498, -0.9845) -> (46.4148, -4.1986)
  line L91 (46.4148, -4.1986) -> (48.2753, -5.6048)
  line L92 (48.2753, -5.6048) -> (46.4663, -7.9981)
  line L93 (46.4663, -7.9981) -> (44.4246, -6.4548)
  line L94 (44.4246, -6.4548) -> (41.4394, -9.8393)
  arc A12 (55, 15) -> (15, 55) centre (15, 15) ccw
  line L95 (15, 55) -> (-15, 55)
  arc A13 (-15, 55) -> (-55, 15) centre (-15, 15) ccw
  line L96 (-55, 15) -> (-55, -15)
  arc A14 (-55, -15) -> (-15, -55) centre (-15, -15) ccw
  line L97 (-15, -55) -> (15, -55)
  arc A15 (15, -55) -> (55, -15) centre (15, -15) ccw
  line L98 (55, -15) -> (55, 15)
  spline S8 degree 3 poles (-36.7171, 17.3686) (-36.8518, 19.0908) (-36.7253, 20.8007) (-35.8249, 23.83) (-35.1927, 25.0859) (-33.575, 27.331) (-32.6362, 28.2988) (-31.607, 29.1577) knots 0.036087 0.036087 0.036087 0.036087 0.555731 0.555731 0.983651 0.983651 1.386095 1.386095 1.386095 1.386095
  line L99 (55, -15) -> (55, 15)
  spline S9 degree 3 poles (10.3534, 38.7474) (11.7335, 39.8031) (13.2103, 40.7051) (16.4323, 41.9003) (18.0613, 42.1653) (21.4266, 42.0265) (23.0731, 41.6295) (26.5653, 40.2029) (28.3145, 39.0547) (30.2985, 37.2379) (30.8783, 36.6163) (31.7024, 35.5077) (32.0008, 35.0361) (32.2468, 34.5387) knots 0.093113 0.093113 0.093113 0.093113 0.616058 0.616058 1.127035 1.127035 1.633478 1.633478 2.269407 2.269407 2.553154 2.553154 2.742163 2.742163 2.742163 2.742163
  arc A16 (-46.5889, -24.0283) -> (-46.959, -29.9997) centre (-47, -27) ccw
  arc A17 (-15, 55) -> (-55, 15) centre (-15, 15) ccw
  arc A18 (55, 15) -> (15, 55) centre (15, 15) ccw
  circle A19 centre (-47, -14) radius 1.5
  arc A20 (-55, -15) -> (-15, -55) centre (-15, -15) ccw
  spline S10 degree 3 poles (-36.7171, 17.3686) (-36.708, 17.2521) (-36.7194, 17.1348) (-36.7821, 16.9096) (-36.833, 16.8034) (-36.901, 16.7084) knots 0 0 0 0 0.035066 0.035066 0.070132 0.070132 0.070132 0.070132
  spline S11 degree 3 poles (26.9165, -31.0417) (26.5017, -31.2521) (26.1072, -31.4995) (24.9398, -32.4102) (24.298, -33.1659) (22.092, -36.2546) (20.5653, -39.283) (15.8311, -43.4069) (14.0247, -44.4113) (11.1819, -45.3972) (9.9898, -45.607) (8.1404, -45.5368) (7.3989, -45.3892) (6.1398, -44.8148) (5.64, -44.4531) (4.7208, -43.4815) (4.3496, -42.8831) (3.4629, -41.0501) (3.1013, -39.695) (2.3137, -37.6472) (1.9455, -36.8825) (1.0366, -35.7978) (0.5937, -35.4393) (-0.469, -34.89) (-1.0783, -34.7097) (-2.9028, -34.4421) (-4.2181, -34.4944) (-5.6597, -34.6622) knots 0.208371 0.208371 0.208371 0.208371 0.359374 0.359374 0.670478 0.670478 1.446599 1.446599 1.895417 1.895417 2.224922 2.224922 2.450473 2.450473 2.63972 2.63972 2.850158 2.850158 3.247941 3.247941 3.519478 3.519478 3.715617 3.715617 3.915643 3.915643 4.242915 4.242915 4.242915 4.242915
  line L100 (-38.3057, 7.5335) -> (-44.436, -2.5576)
  spline S12 degree 3 poles (-26.7602, -29.7249) (-26.63, -29.7231) (-26.5007, -29.7468) (-26.2585, -29.8424) (-26.1478, -29.9134) (-25.9828, -30.072) (-25.9221, -30.1505) (-25.8258, -30.3228) (-25.7906, -30.4155) (-25.7696, -30.512) knots 0 0 0 0 0.039064 0.039064 0.078129 0.078129 0.107731 0.107731 0.137333 0.137333 0.137333 0.137333
  line L101 (-6.2674, -36.346) -> (-5.7671, -36.87)
  circle A21 centre (47, -22) radius 1.5
  line L102 (15, 55) -> (-15, 55)
  circle A22 centre (-47.207, 20.5835) radius 1.5
  circle A23 centre (-21.042, -45.9567) radius 1.5
  line L103 (-55, 15) -> (-55, -15)
  spline S13 degree 3 poles (-26.1708, -25.1385) (-26.1038, -20.834) (-25.4712, -16.205) (-26.5447, -7.6817) (-27.7362, -4.5994) (-31.188, 2.4366) (-33.2656, 6.0733) (-34.7718, 9.827) knots 0.104133 0.104133 0.104133 0.104133 1.379101 1.379101 2.416171 2.416171 3.406243 3.406243 3.406243 3.406243
  line L104 (-15, -55) -> (15, -55)
  spline S14 degree 3 poles (-25.443, 32.8404) (-22.6391, 34.0489) (-19.6406, 34.8647) (-13.9908, 35.6095) (-11.9033, 35.3478) (-8.6393, 34.4929) (-7.241, 33.737) (-4.6779, 32.215) (-3.539, 31.4712) (-1.7666, 30.8258) (-1.1355, 30.6903) (0.1203, 30.7222) (0.6844, 30.8607) (1.9595, 31.399) (2.6674, 31.8714) (4.1765, 33.0867) (4.9824, 33.8527) (5.8326, 34.6756) knots 0.182197 0.182197 0.182197 0.182197 1.090679 1.090679 2.116632 2.116632 3.315493 3.315493 4.459674 4.459674 5.071625 5.071625 5.626071 5.626071 6.359803 6.359803 7.157958 7.157958 7.157958 7.157958
  spline S15 degree 3 poles (33.0286, 28.0718) (33.0703, 27.3997) (33.1676, 26.6977) (33.5348, 25.6326) (33.7207, 25.3268) (34.1024, 24.8702) (34.3236, 24.7044) (34.8418, 24.4372) (35.1527, 24.347) (36.4443, 24.0711) (37.7665, 23.9707) (40.2586, 22.8614) (41.1591, 22.2488) (42.5804, 20.7638) (43.1055, 19.9446) (43.8206, 18.0888) (43.9818, 17.0988) (44.0027, 14.699) (43.7263, 13.2998) (42.5231, 9.2938) (41.1447, 6.638) (39.093, 2.0196) (38.3333, 0.1029) (37.4451, -3.4515) (37.2198, -4.8242) (37.0928, -6.2158) knots 0.129203 0.129203 0.129203 0.129203 0.294006 0.294006 0.417435 0.417435 0.550082 0.550082 0.704478 0.704478 1.129194 1.129194 1.408869 1.408869 1.66214 1.66214 1.922723 1.922723 2.2812 2.2812 3.001747 3.001747 3.492602 3.492602 3.809237 3.809237 3.809237 3.809237
  circle A24 centre (19.8064, 49.2459) radius 1.5
  spline S16 degree 3 poles (10.3534, 38.7474) (10.25, 38.6683) (10.1321, 38.6101) (9.8807, 38.5423) (9.7495, 38.5332) (9.501, 38.5647) (9.3853, 38.6012) (9.1724, 38.7136) (9.077, 38.7886) (8.9972, 38.8787) knots 0 0 0 0 0.039064 0.039064 0.078129 0.078129 0.114234 0.114234 0.150339 0.150339 0.150339 0.150339
  line L105 (-5.7671, -36.87) -> (3.0074, -44.7706)
  circle A25 centre (-38.15, -37.75) radius 2.75
  spline S17 degree 3 poles (-12.6849, -35.825) (-15.1523, -36.2299) (-17.5661, -36.5071) (-20.6177, -36.1408) (-21.5954, -35.8949) (-23.1516, -35.0659) (-23.7332, -34.592) (-24.6878, -33.4235) (-25.0394, -32.7732) (-25.5022, -31.577) (-25.6531, -31.0471) (-25.7696, -30.512) knots 0.057698 0.057698 0.057698 0.057698 0.810588 0.810588 1.168868 1.168868 1.446193 1.446193 1.71283 1.71283 1.908956 1.908956 1.908956 1.908956
  line L106 (32.8215, 34.0352) -> (36.3135, 32.8488)
  line L107 (5.8857, 36.0571) -> (5.3836, 36.6241)
  line L108 (-49.3002, 0.9259) -> (-41.7204, 9.9789)
  line L109 (-31.2503, 29.8533) -> (-30.8456, 35.4405)
  circle A26 centre (-14, 47) radius 1.5
  spline S18 degree 3 poles (33.0286, 28.0718) (33.0205, 28.2018) (33.0379, 28.3321) (33.1217, 28.5787) (33.1873, 28.6926) (33.3584, 28.889) (33.4623, 28.9695) (33.6951, 29.0862) (33.8218, 29.1212) (34.0186, 29.136) (34.0859, 29.1343) (34.2192, 29.1174) (34.2848, 29.1022) (34.3484, 29.0806) knots 0 0 0 0 0.039064 0.039064 0.078129 0.078129 0.117193 0.117193 0.156258 0.156258 0.176407 0.176407 0.196555 0.196555 0.196555 0.196555
  line L110 (24.1405, -46.0928) -> (27.7111, -34.8384)
  spline S19 degree 3 poles (-26.1708, -25.1385) (-26.1728, -25.2687) (-26.2002, -25.3972) (-26.3028, -25.6366) (-26.377, -25.7451) (-26.5628, -25.9276) (-26.6727, -25.9998) (-26.8626, -26.0772) (-26.9349, -26.0976) (-27.0827, -26.1219) (-27.1577, -26.1256) (-27.2325, -26.121) knots 0 0 0 0 0.039064 0.039064 0.078129 0.078129 0.117193 0.117193 0.139661 0.139661 0.162129 0.162129 0.162129 0.162129
  arc A27 (1.3897, 48.8137) -> (-3.0893, 44.8472) centre (-1, 47) ccw
  line L111 (-36.5129, 10.0369) -> (-38.3057, 7.5335)
  spline S20 degree 3 poles (-12.6849, -35.825) (-12.5564, -35.8039) (-12.425, -35.8081) (-12.1912, -35.8621) (-12.0889, -35.9043) (-11.9023, -36.0201) (-11.8192, -36.093) (-11.7496, -36.1779) knots 0 0 0 0 0.039064 0.039064 0.072008 0.072008 0.104952 0.104952 0.104952 0.104952
  arc A28 (24.1405, -46.0928) -> (29.9635, -47.4663) centre (27, -47) ccw
  line L112 (-26.7602, -29.7249) -> (-35.1529, -29.8382)
  arc A29 (-1.3202, -48.9018) -> (3.0074, -44.7706) centre (1, -47) ccw
  spline S21 degree 3 poles (26.9165, -31.0417) (27.0327, -30.9828) (27.1592, -30.9471) (27.4188, -30.9264) (27.5494, -30.9414) (27.7975, -31.0207) (27.9125, -31.0842) (28.1119, -31.2518) (28.1943, -31.3542) (28.3101, -31.5753) (28.3461, -31.6901) (28.3759, -31.9269) (28.3695, -32.047) (28.3421, -32.1631) knots 0 0 0 0 0.039064 0.039064 0.078129 0.078129 0.117193 0.117193 0.156258 0.156258 0.192058 0.192058 0.227858 0.227858 0.227858 0.227858
  spline S22 degree 3 poles (38.0888, -7.3067) (37.9586, -7.3067) (37.8296, -7.2813) (37.5887, -7.1825) (37.479, -7.11) (37.2936, -6.9271) (37.2197, -6.8184) (37.1364, -6.6228) (37.1136, -6.5433) (37.088, -6.3805) (37.0853, -6.2979) (37.0928, -6.2158) knots 0 0 0 0 0.039064 0.039064 0.078129 0.078129 0.117193 0.117193 0.141909 0.141909 0.166624 0.166624 0.166624 0.166624
  spline S23 degree 3 poles (32.8215, 34.0352) (32.6982, 34.0771) (32.5843, 34.1427) (32.3866, 34.3149) (32.3053, 34.4205) (32.2468, 34.5387) knots 0 0 0 0 0.039064 0.039064 0.078649 0.078649 0.078649 0.078649
  arc A30 (49.2498, -0.9845) -> (44.477, 2.6231) centre (47, 1) ccw
  arc A31 (45.8232, 24.2404) -> (47.7479, 29.9053) centre (47, 27) ccw
  circle A32 centre (37.75, -38.15) radius 2.75
  spline S24 degree 3 poles (37.3555, -15.6808) (37.7175, -19.3956) (38.116, -22.8083) (37.3203, -26.0559) (37.037, -26.7219) (36.2871, -27.772) (35.8641, -28.165) (34.7771, -28.8627) (34.1119, -29.1251) (33.3998, -29.3308) knots 0.039171 0.039171 0.039171 0.039171 1.164828 1.164828 1.516946 1.516946 1.81941 1.81941 2.171391 2.171391 2.171391 2.171391
  line L113 (27.7111, -34.8384) -> (28.3421, -32.1631)
  circle A33 centre (14, -47) radius 1.5
  circle A34 centre (38.15, 37.75) radius 2.75
  line L114 (31.7989, -35.8027) -> (29.9635, -47.4663)
  spline S25 degree 3 poles (37.3555, -15.6808) (37.3434, -15.557) (37.3546, -15.432) (37.4222, -15.1925) (37.478, -15.0801) (37.553, -14.9808) knots 0 0 0 0 0.037327 0.037327 0.074653 0.074653 0.074653 0.074653
  spline S26 degree 3 poles (32.6895, -30.1363) (32.7097, -30.0076) (32.7548, -29.8842) (32.8899, -29.6615) (32.9786, -29.5645) (33.1787, -29.4167) (33.2859, -29.3637) (33.3998, -29.3308) knots 0 0 0 0 0.039064 0.039064 0.078129 0.078129 0.113706 0.113706 0.113706 0.113706
  line L115 (32.6895, -30.1363) -> (31.7989, -35.8027)
  line L116 (41.4394, -9.8393) -> (37.553, -14.9808)
  line L117 (49.2498, -0.9845) -> (41.4394, -9.8393)
  line L118 (38.0888, -7.3067) -> (44.477, 2.6231)
  line L119 (-34.8931, -25.6463) -> (-27.2325, -26.121)
  circle A35 centre (47, 14) radius 1.5
  line L120 (-41.7204, 9.9789) -> (-36.901, 16.7084)
  spline S27 degree 3 poles (-36.5129, 10.0369) (-36.4371, 10.1428) (-36.3413, 10.2328) (-36.1206, 10.3711) (-35.9978, 10.4181) (-35.7412, 10.4622) (-35.6098, 10.4591) (-35.3556, 10.4025) (-35.2352, 10.3497) (-35.0488, 10.2198) (-34.9777, 10.1531) (-34.8569, 10.0013) (-34.8079, 9.917) (-34.7718, 9.827) knots 0 0 0 0 0.039064 0.039064 0.078129 0.078129 0.117193 0.117193 0.156258 0.156258 0.185351 0.185351 0.214445 0.214445 0.214445 0.214445
  line L121 (-1.3202, -48.9018) -> (-11.7496, -36.1779)
  spline S28 degree 3 poles (5.8857, 36.0571) (5.9721, 35.9596) (6.0385, 35.8462) (6.1242, 35.6003) (6.1427, 35.4702) (6.1286, 35.2101) (6.0962, 35.0827) (5.989, 34.8569) (5.9186, 34.7589) (5.8326, 34.6756) knots 0 0 0 0 0.039064 0.039064 0.078129 0.078129 0.117193 0.117193 0.153113 0.153113 0.153113 0.153113
  line L122 (-30.8456, 35.4405) -> (-29.9922, 47.2169)
  line L123 (5.3836, 36.6241) -> (-3.0893, 44.8472)
  spline S29 degree 3 poles (-25.443, 32.8404) (-25.5626, 32.7889) (-25.6911, 32.7612) (-25.9515, 32.7567) (-26.0809, 32.7798) (-26.3235, 32.8745) (-26.4344, 32.945) (-26.623, 33.1247) (-26.6988, 33.2321) (-26.7905, 33.4375) (-26.8167, 33.5292) (-26.8424, 33.7171) (-26.8419, 33.8124) (-26.8279, 33.9062) knots 0 0 0 0 0.039064 0.039064 0.078129 0.078129 0.117193 0.117193 0.156258 0.156258 0.184704 0.184704 0.21315 0.21315 0.21315 0.21315
  line L124 (36.3135, 32.8488) -> (47.7479, 29.9053)
  arc A36 (-24.0746, 46.3351) -> (-29.9922, 47.2169) centre (-27, 47) ccw
  line L125 (-24.0746, 46.3351) -> (-26.6915, 34.8215)
  line L126 (1.3897, 48.8137) -> (8.5279, 39.4086)
  line L127 (-46.5889, -24.0283) -> (-34.8931, -25.6463)
  line L128 (45.8232, 24.2404) -> (34.9623, 28.872)
  spline S30 degree 3 poles (-31.2503, 29.8533) (-31.2597, 29.7234) (-31.2944, 29.5966) (-31.3831, 29.4182) (-31.4202, 29.3598) (-31.5057, 29.2515) (-31.554, 29.2019) (-31.607, 29.1577) knots 0 0 0 0 0.039064 0.039064 0.059766 0.059766 0.080467 0.080467 0.080467 0.080467
  arc A37 (-49.3002, 0.9259) -> (-44.436, -2.5576) centre (-47, -1) ccw
  spline S31 degree 3 poles (-6.2674, -36.346) (-6.3573, -36.2519) (-6.4279, -36.141) (-6.5228, -35.8985) (-6.5461, -35.7691) (-6.5417, -35.5087) (-6.5142, -35.3802) (-6.4113, -35.1409) (-6.337, -35.0325) (-6.1653, -34.8642) (-6.0744, -34.8007) (-5.8756, -34.7057) (-5.7691, -34.675) (-5.6597, -34.6622) knots 0 0 0 0 0.039064 0.039064 0.078129 0.078129 0.117193 0.117193 0.156258 0.156258 0.189303 0.189303 0.222349 0.222349 0.222349 0.222349
  line L129 (-35.1529, -29.8382) -> (-46.959, -29.9997)
  circle A38 centre (-37.75, 38.15) radius 2.75
  arc A39 (15, -55) -> (55, -15) centre (15, -15) ccw
  line L130 (-26.6915, 34.8215) -> (-26.8279, 33.9062)
  line L131 (34.9623, 28.872) -> (34.3484, 29.0806)
  line L132 (8.5279, 39.4086) -> (8.9972, 38.8787)
  circle A40 centre (-38.15, -37.75) radius 1.25
  circle A41 centre (37.75, -38.15) radius 1.25
  circle A42 centre (38.15, 37.75) radius 1.25
  circle A43 centre (-37.75, 38.15) radius 1.25
  dimension "d125" = 3
  dimension "d126" = 3
  dimension "d127" = 3